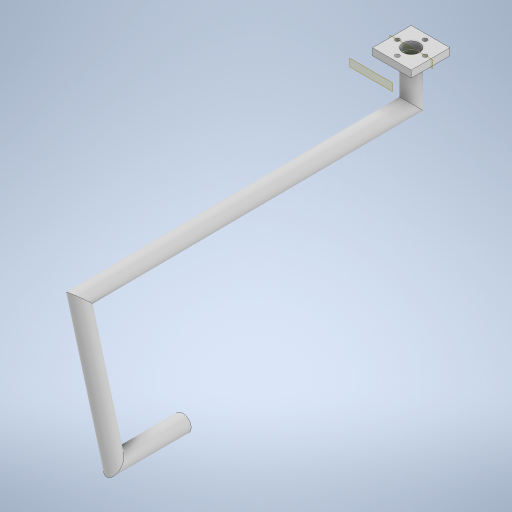
# Autodesk Inventor part: water tube to pump
Saved by Autodesk Inventor 2023 (Build 270158000, 158)
## iProperties
Created: 2022-11-25
Part Number: water tube to pump
Material: Generic
Document SubType Name: Modeling
Designer: hp
Density: 1 g/cm^3
Appearance: Default
Author: hp
Autodesk Inventor part; units mm, degrees
ref_plane "YZ Plane" through (0, 0, 0) normal (1, 0, 0) x (0, 1, 0)
ref_plane "XZ Plane" through (0, 0, 0) normal (0, 1, 0) x (-1, 0, 0)
ref_plane "XY Plane" through (0, 0, 0) normal (0, 0, 1) x (1, 0, 0)
sketch "Sketch1" plane through (0, 0, 0) normal (0, 1, 0) x (-1, 0, 0)
  line L0 (14, 14) -> (-14, 14)
  line L1 (-14, 14) -> (-14, -14)
  line L2 (-14, -14) -> (14, -14)
  line L3 (14, -14) -> (14, 14)
  point P0 (0, 0)
  point P1 (0, -14)
  dimension "d0" = 28
  dimension "d1" = 28
  dimension "d2" = 14
  dimension "d3" = 14
  constraints: 8 end point, 2 parallel, 1 horizontal, 1 midpoint, 1 perpendicular
  measures "d0" distance of L2.end L0.start
  measures "d1" distance of L1.end L2.end
  measures "d2" distance of point (0, -14) point (0, 0)
  measures "d3" distance from line of L1 point (0, 0)
extrude "Extrusion1" add sketch "Sketch1" along normal blind 5
sketch "Sketch2" plane through (0, 5, 0) normal (0, 1, 0) x (1, 0, 0)
  circle A0 centre (0, 0) radius 6
  circle A1 centre (-10, 0) radius 1.5
  circle A2 centre (0, -10) radius 1.5
  circle A3 centre (10, 0) radius 1.5
  circle A4 centre (0, 10) radius 1.5
  dimension "d6" = 12
  dimension "d7" = 3
  dimension "d8" = 10
  dimension "d11" = 360
  constraints: 5 centre point, 1 coincident, 9 other
  measures "d6" diameter of A0
  measures "d7" diameter of A1
  measures "d8" distance of A0.centre A1.centre
extrude "Extrusion2" cut sketch "Sketch2" against normal blind 5
ref_plane "Work Plane1" through (14, 0, 0) normal (0, 0, -1) x (-1, 0, 0)
sketch "Sketch3" plane through (14, 0, 0) normal (0, 0, -1) x (-1, 0, 0)
  point P0 (14, 0)
sketch "Sketch4" plane through (0, 0, 0) normal (0, -1, 0) x (1, 0, 0)
  circle A0 centre (0, 0) radius 6
  circle A1 centre (0, 0) radius 5
  dimension "d19" = 10
  dimension "d22" = 12
  constraints: 2 centre point, 2 coincident
  measures "d19" diameter of A1
  measures "d22" diameter of A0
sketch3d "3D Sketch1"
  line L0 (0, 0, 0) -> (0, -30, 0)
  line L1 (0, -30, 0) -> (0, -31.7049, 239.9939)
  line L2 (0, -31.7049, 239.9939) -> (17.3648, -129.9033, 232.5414)
  line L3 (17.3648, -129.9033, 232.5414) -> (17.3648, -129.9033, 182.5414)
  dimension "d16" = 30
  dimension "d53" = 100
  dimension "d54" = 80
  dimension "d55" = 50
  dimension "d56" = 240
  dimension "d57" = 90
sweep "Sweep1" add profiles "Sketch4" path "3D Sketch1"
chamfer "Chamfer1" distance 1 angle 45 4 edges at (8.5, 0, 0) (-1.5, 0, 10) (-1.5, 0, -10) (-11.5, 0, 0)
ref_plane "Work Plane2" through (-14, 0, 29) normal (0, 0, 1) x (1, 0, 0)
body "Solid1"
